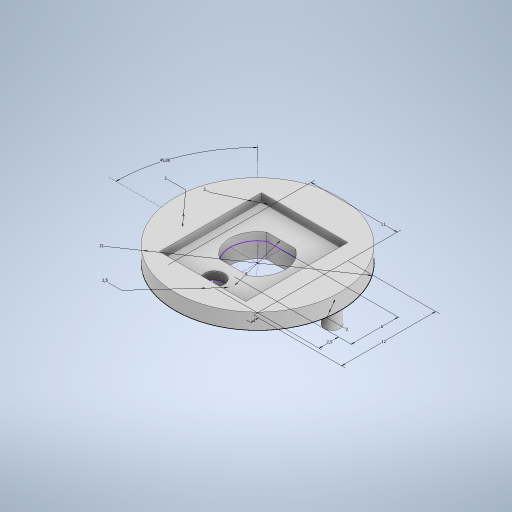
# Autodesk Inventor part: Switch1
Saved by Autodesk Inventor 2024 (Build 280153000, 153)
## iProperties
Created: 2023-06-19
Part Number: Switch1
Material: Типовые
Document SubType Name: Modeling
Designer: fm
Density: 1 g/cm^3
Appearance: По умолчанию
Author: fm
Autodesk Inventor part; units mm, degrees
ref_plane "YZ Plane" through (0, 0, 0) normal (1, 0, 0) x (0, 1, 0)
ref_plane "XZ Plane" through (0, 0, 0) normal (0, 1, 0) x (-1, 0, 0)
ref_plane "XY Plane" through (0, 0, 0) normal (0, 0, 1) x (1, 0, 0)
sketch "Эскиз1" plane through (0, 0, 0) normal (0, 1, 0) x (-1, 0, 0)
  circle A0 centre (0, 0) radius 10.5
  circle A1 centre (0, 0) radius 4
  line L0 (0, -3) -> (0, 3) construction
  line L1 (1.8028, -3) -> (-1.8028, -3)
  line L2 (-1.8028, 3) -> (1.8028, 3)
  circle A2 centre (0, 5.5) radius 1.25
  circle A3 centre (9.5, 0) radius 1
  circle A4 centre (-9.5, 0) radius 1
  line L3 (5.5, -6) -> (-5.5, -6)
  line L4 (-5.5, -6) -> (-5.5, 6)
  line L5 (5.5, 6) -> (5.5, -6)
  line L6 (5.5, -6) -> (-5.5, 6) construction
  line L7 (0, 10.5) -> (0, -10.5) construction
  arc A5 (1.8028, -3) -> (1.8028, 3) centre (0, 0) ccw
  arc A6 (-1.8028, 3) -> (-1.8028, -3) centre (0, 0) ccw
  arc A7 (1.8028, -3) -> (1.8028, 3) centre (0, 0) ccw
  arc A8 (-1.8028, 3) -> (-1.8028, -3) centre (0, 0) ccw
  line L8 (-5.5, 6) -> (-1.1456, 6)
  line L9 (1.1456, 6) -> (5.5, 6)
  line L10 (5.5, 6) -> (-5.5, 6)
  line L11 (-5.5, 6) -> (-5.5, 7)
  line L12 (-5.5, 7) -> (5.5, 7)
  line L13 (5.5, 7) -> (5.5, 6)
  line L14 (11.1303, -11.1303) -> (0, 0) construction
  line L15 (0, 0) -> (18.9619, 0) construction
  circle A9 centre (6.7175, -6.7175) radius 1
  dimension "d0" = 21
  dimension "d1" = 8
  dimension "d3" = 6
  dimension "d4" = 2.5
  dimension "d5" = 2.5
  dimension "d6" = 2
  dimension "d7" = 2
  dimension "d8" = 11
  dimension "d9" = 12
  dimension "d18" = 1
  dimension "d21" = 45
  dimension "d22" = 2
  constraints: 32 end point, 12 point on circle, 10 centre point, 7 coincident, 5 parallel, 4 horizontal, 4 midpoint, 3 tangent, 2 perpendicular, 1 point on line, 1 vertical
  measures "d0" diameter of A0
  measures "d1" diameter of A1
  measures "d3" distance of L0.start L0.end
  measures "d4" diameter of A2
  measures "d5" distance from line of A2.centre L2
  measures "d6" diameter of A3
  measures "d7" diameter of A4
  measures "d8" distance of L4.end L5.start
  measures "d9" distance of L3.end L4.end
  measures "d18" distance of L10.end L11.end
  measures "d21" angle of L15 L14
  measures "d22" diameter of A9
extrude "Выдавливание1" add sketch "Эскиз1" along normal blind 1 contours A4 | A9 | A0 | A3 | A1 | A2 L9 L5 L3 L4 L8 | A2 L8 L11 L12 L13 L9
extrude "Выдавливание2" add sketch "Эскиз1" along normal blind 1 from surface at 1 contours A4 | A9 | A0 | A3 | A2 L8 L11 L12 L13 L9
extrude "Выдавливание3" add sketch "Эскиз1" against normal blind 2 contours A1
extrude "Выдавливание4" add sketch "Эскиз1" against normal blind 2 contours A4 | A3
extrude "Выдавливание5" cut sketch "Эскиз1" against normal up to surface (1 mm away) from surface at 2 contours A2 L8 L11 L12 L13 L9
extrude "Выдавливание6" add sketch "Эскиз1" against normal blind 2 contours A9
